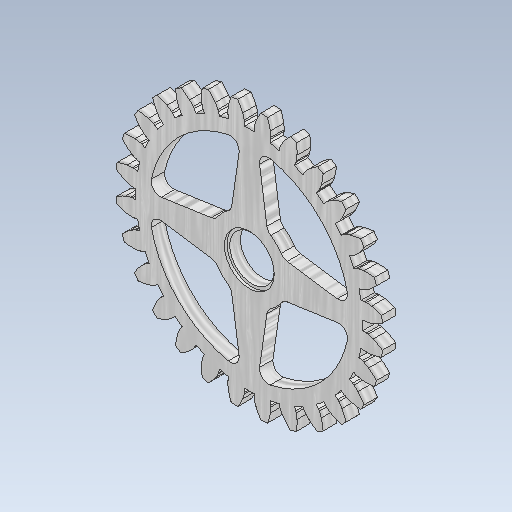
# Autodesk Inventor part: ｍ2歯数28ギア改二d10
Saved by Autodesk Inventor 2020.2 (Build 242310000, 310)
## iProperties
Created: 2020-02-11
Part Number: ｍ2歯数28ギア改二d10
Material: アルミニウム 7075
Document SubType Name: Modeling
Designer: aoyam
Density: 2.81 g/cm^3
Appearance: サテン - ブラシ仕上げ 重厚
Author: aoyam
Autodesk Inventor part; units mm, degrees
ref_plane "YZ Plane" through (0, 0, 0) normal (1, 0, 0) x (0, 1, 0)
ref_plane "XZ Plane" through (0, 0, 0) normal (0, 1, 0) x (-1, 0, 0)
ref_plane "XY Plane" through (0, 0, 0) normal (0, 0, 1) x (1, 0, 0)
sketch "スケッチ1" plane through (0, 0, 0) normal (0, 0, 1) x (1, 0, 0)
  arc A0 (149.6408, 131.6584) -> (149.5836, 131.2891) centre (152.0659, 131.0938) ccw
  arc A1 (150.0089, 132.8103) -> (149.6408, 131.6584) centre (156.3128, 130.1608) ccw
  arc A2 (151.1316, 134.8844) -> (150.0089, 132.8103) centre (160.8866, 128.2633) ccw
  arc A3 (147.4164, 131.2891) -> (147.3592, 131.6584) centre (144.9341, 131.0938) ccw
  arc A4 (147.3592, 131.6584) -> (146.9911, 132.8103) centre (140.6872, 130.1608) ccw
  arc A5 (146.9911, 132.8103) -> (145.8684, 134.8844) centre (136.1134, 128.2633) ccw
  arc A6 (149.5502, 130.4784) -> (147.4498, 130.4784) centre (148.5, 105) ccw
  arc A7 (145.8684, 134.8844) -> (144.4157, 134.7207) centre (148.5, 105) ccw
  line L0 (149.5502, 130.4784) -> (149.5836, 131.2891)
  line L1 (147.4498, 130.4784) -> (147.4164, 131.2891)
  line L2 (116.5, 105) -> (180.5, 105)
  line L3 (148.5, 73) -> (148.5, 137)
  line L4 (198.5, 135) -> (268.5, 135)
  line L5 (198.5, 127) -> (268.5, 127)
  line L6 (198.5, 119) -> (268.5, 119)
  line L7 (198.5, 111) -> (268.5, 111)
  line L8 (198.5, 103) -> (268.5, 103)
  line L9 (198.5, 95) -> (268.5, 95)
  line L10 (198.5, 87) -> (268.5, 87)
  line L11 (198.5, 79) -> (268.5, 79)
  line L12 (198.5, 71) -> (268.5, 71)
  line L13 (198.5, 63) -> (268.5, 63)
  line L14 (198.5, 55) -> (268.5, 55)
  line L15 (198.5, 47) -> (268.5, 47)
  line L16 (198.5, 39) -> (268.5, 39)
  line L17 (198.5, 135) -> (198.5, 39)
  line L18 (268.5, 135) -> (268.5, 39)
  line L19 (233.5, 127) -> (233.5, 39)
  arc A8 (144.4157, 134.7207) -> (143.7827, 132.4488) centre (155.3995, 130.4363) ccw
  arc A9 (143.7827, 132.4488) -> (143.6801, 131.2439) centre (150.5181, 131.2684) ccw
  arc A10 (143.6801, 131.2439) -> (143.7066, 130.8711) centre (146.1701, 131.2331) ccw
  line L20 (143.8544, 130.0733) -> (143.7066, 130.8711)
  arc A11 (143.8544, 130.0733) -> (141.8067, 129.6059) centre (148.5, 105) ccw
  line L21 (141.8067, 129.6059) -> (141.5937, 130.3888)
  arc A12 (141.5937, 130.3888) -> (141.4558, 130.7362) centre (139.217, 129.6461) ccw
  arc A13 (141.4558, 130.7362) -> (140.8405, 131.7773) centre (135.2843, 127.7914) ccw
  arc A14 (140.8405, 131.7773) -> (139.2845, 133.5495) centre (131.2474, 124.9238) ccw
  arc A15 (139.2845, 133.5495) -> (137.9046, 133.0667) centre (148.5, 105) ccw
  arc A16 (137.9046, 133.0667) -> (137.7931, 130.7109) centre (149.5664, 131.3339) ccw
  arc A17 (137.7931, 130.7109) -> (137.9612, 129.5133) centre (144.6222, 131.0589) ccw
  arc A18 (137.9612, 129.5133) -> (138.0699, 129.1558) centre (140.3911, 130.0569) ccw
  line L22 (138.3915, 128.4109) -> (138.0699, 129.1558)
  arc A19 (138.3915, 128.4109) -> (136.4992, 127.4996) centre (148.5, 105) ccw
  line L23 (136.4992, 127.4996) -> (136.1173, 128.2155)
  arc A20 (136.1173, 128.2155) -> (135.9056, 128.5234) centre (133.9655, 126.9625) ccw
  arc A21 (135.9056, 128.5234) -> (135.0741, 129.4015) centre (130.5441, 124.2792) ccw
  arc A22 (135.0741, 129.4015) -> (133.1627, 130.7831) centre (127.2465, 120.5852) ccw
  arc A23 (133.1627, 130.7831) -> (131.9249, 130.0053) centre (148.5, 105) ccw
  arc A24 (131.9249, 130.0053) -> (132.3403, 127.6838) centre (143.6798, 130.9109) ccw
  arc A25 (132.3403, 127.6838) -> (132.7707, 126.5536) centre (138.9208, 129.5427) ccw
  arc A26 (132.7707, 126.5536) -> (132.9562, 126.2292) centre (135.0187, 127.6243) ccw
  line L24 (133.4356, 125.5746) -> (132.9562, 126.2292)
  arc A27 (133.4356, 125.5746) -> (131.7934, 124.265) centre (148.5, 105) ccw
  line L25 (131.7934, 124.265) -> (131.2618, 124.878)
  arc A28 (131.2618, 124.878) -> (130.9869, 125.1311) centre (129.4428, 123.1776) ccw
  arc A29 (130.9869, 125.1311) -> (129.9808, 125.8022) centre (126.7042, 119.8003) ccw
  arc A30 (129.9808, 125.8022) -> (127.81, 126.7238) centre (124.3113, 115.4651) ccw
  arc A31 (127.81, 126.7238) -> (126.7762, 125.69) centre (148.5, 105) ccw
  arc A32 (126.7762, 125.69) -> (127.6978, 123.5192) centre (138.0349, 129.1887) ccw
  arc A33 (127.6978, 123.5192) -> (128.3689, 122.5131) centre (133.6997, 126.7958) ccw
  arc A34 (128.3689, 122.5131) -> (128.622, 122.2382) centre (130.3224, 124.0572) ccw
  line L26 (129.235, 121.7066) -> (128.622, 122.2382)
  arc A35 (129.235, 121.7066) -> (127.9254, 120.0644) centre (148.5, 105) ccw
  line L27 (127.9254, 120.0644) -> (127.2708, 120.5438)
  arc A36 (127.2708, 120.5438) -> (126.9464, 120.7293) centre (125.8757, 118.4813) ccw
  arc A37 (126.9464, 120.7293) -> (125.8162, 121.1597) centre (123.9573, 114.5792) ccw
  arc A38 (125.8162, 121.1597) -> (123.4947, 121.5751) centre (122.5891, 109.8202) ccw
  arc A39 (123.4947, 121.5751) -> (122.7169, 120.3373) centre (148.5, 105) ccw
  arc A40 (122.7169, 120.3373) -> (124.0985, 118.4259) centre (132.9148, 126.2535) ccw
  arc A41 (124.0985, 118.4259) -> (124.9766, 117.5944) centre (129.2208, 122.9559) ccw
  arc A42 (124.9766, 117.5944) -> (125.2845, 117.3827) centre (126.5375, 119.5345) ccw
  line L28 (126.0004, 117.0008) -> (125.2845, 117.3827)
  arc A43 (126.0004, 117.0008) -> (125.0891, 115.1085) centre (148.5, 105) ccw
  line L29 (125.0891, 115.1085) -> (124.3442, 115.4301)
  arc A44 (124.3442, 115.4301) -> (123.9867, 115.5388) centre (123.4431, 113.1089) ccw
  arc A45 (123.9867, 115.5388) -> (122.7891, 115.7069) centre (122.4411, 108.8778) ccw
  arc A46 (122.7891, 115.7069) -> (120.4333, 115.5954) centre (122.1661, 103.9336) ccw
  arc A47 (120.4333, 115.5954) -> (119.9505, 114.2155) centre (148.5, 105) ccw
  arc A48 (119.9505, 114.2155) -> (121.7227, 112.6595) centre (128.5762, 122.2526) ccw
  arc A49 (121.7227, 112.6595) -> (122.7638, 112.0442) centre (125.7086, 118.2157) ccw
  arc A50 (122.7638, 112.0442) -> (123.1112, 111.9063) centre (123.8539, 114.283) ccw
  line L30 (123.8941, 111.6933) -> (123.1112, 111.9063)
  arc A51 (123.8941, 111.6933) -> (123.4267, 109.6456) centre (148.5, 105) ccw
  line L31 (123.4267, 109.6456) -> (122.6289, 109.7934)
  arc A52 (122.6289, 109.7934) -> (122.2561, 109.8199) centre (122.2669, 107.3299) ccw
  arc A53 (122.2561, 109.8199) -> (121.0512, 109.7173) centre (122.2316, 102.9819) ccw
  arc A54 (121.0512, 109.7173) -> (118.7793, 109.0843) centre (123.0637, 98.1005) ccw
  arc A55 (118.7793, 109.0843) -> (118.6156, 107.6316) centre (148.5, 105) ccw
  arc A56 (118.6156, 107.6316) -> (120.6897, 106.5089) centre (125.2367, 117.3866) ccw
  arc A57 (120.6897, 106.5089) -> (121.8416, 106.1408) centre (123.3392, 112.8128) ccw
  arc A58 (121.8416, 106.1408) -> (122.2109, 106.0836) centre (122.4062, 108.5659) ccw
  line L32 (123.0216, 106.0502) -> (122.2109, 106.0836)
  arc A59 (123.0216, 106.0502) -> (123.0216, 103.9498) centre (148.5, 105) ccw
  line L33 (123.0216, 103.9498) -> (122.2109, 103.9164)
  arc A60 (122.2109, 103.9164) -> (121.8416, 103.8592) centre (122.4062, 101.4341) ccw
  arc A61 (121.8416, 103.8592) -> (120.6897, 103.4911) centre (123.3392, 97.1872) ccw
  arc A62 (120.6897, 103.4911) -> (118.6156, 102.3684) centre (125.2367, 92.6134) ccw
  arc A63 (118.6156, 102.3684) -> (118.7793, 100.9157) centre (148.5, 105) ccw
  arc A64 (118.7793, 100.9157) -> (121.0512, 100.2827) centre (123.0637, 111.8995) ccw
  arc A65 (121.0512, 100.2827) -> (122.2561, 100.1801) centre (122.2316, 107.0181) ccw
  arc A66 (122.2561, 100.1801) -> (122.6289, 100.2066) centre (122.2669, 102.6701) ccw
  line L34 (123.4267, 100.3544) -> (122.6289, 100.2066)
  arc A67 (123.4267, 100.3544) -> (123.8941, 98.3067) centre (148.5, 105) ccw
  line L35 (123.8941, 98.3067) -> (123.1112, 98.0937)
  arc A68 (123.1112, 98.0937) -> (122.7638, 97.9558) centre (123.8539, 95.717) ccw
  arc A69 (122.7638, 97.9558) -> (121.7227, 97.3405) centre (125.7086, 91.7843) ccw
  arc A70 (121.7227, 97.3405) -> (119.9505, 95.7845) centre (128.5762, 87.7474) ccw
  arc A71 (119.9505, 95.7845) -> (120.4333, 94.4046) centre (148.5, 105) ccw
  arc A72 (120.4333, 94.4046) -> (122.7891, 94.2931) centre (122.1661, 106.0664) ccw
  arc A73 (122.7891, 94.2931) -> (123.9867, 94.4612) centre (122.4411, 101.1222) ccw
  arc A74 (123.9867, 94.4612) -> (124.3442, 94.5699) centre (123.4431, 96.8911) ccw
  line L36 (125.0891, 94.8915) -> (124.3442, 94.5699)
  arc A75 (125.0891, 94.8915) -> (126.0004, 92.9992) centre (148.5, 105) ccw
  line L37 (126.0004, 92.9992) -> (125.2845, 92.6173)
  arc A76 (125.2845, 92.6173) -> (124.9766, 92.4056) centre (126.5375, 90.4655) ccw
  arc A77 (124.9766, 92.4056) -> (124.0985, 91.5741) centre (129.2208, 87.0441) ccw
  arc A78 (124.0985, 91.5741) -> (122.7169, 89.6627) centre (132.9148, 83.7465) ccw
  arc A79 (122.7169, 89.6627) -> (123.4947, 88.4249) centre (148.5, 105) ccw
  arc A80 (123.4947, 88.4249) -> (125.8162, 88.8403) centre (122.5891, 100.1798) ccw
  arc A81 (125.8162, 88.8403) -> (126.9464, 89.2707) centre (123.9573, 95.4208) ccw
  arc A82 (126.9464, 89.2707) -> (127.2708, 89.4562) centre (125.8757, 91.5187) ccw
  line L38 (127.9254, 89.9356) -> (127.2708, 89.4562)
  arc A83 (127.9254, 89.9356) -> (129.235, 88.2934) centre (148.5, 105) ccw
  line L39 (129.235, 88.2934) -> (128.622, 87.7618)
  arc A84 (128.622, 87.7618) -> (128.3689, 87.4869) centre (130.3224, 85.9428) ccw
  arc A85 (128.3689, 87.4869) -> (127.6978, 86.4808) centre (133.6997, 83.2042) ccw
  arc A86 (127.6978, 86.4808) -> (126.7762, 84.31) centre (138.0349, 80.8113) ccw
  arc A87 (126.7762, 84.31) -> (127.81, 83.2762) centre (148.5, 105) ccw
  arc A88 (127.81, 83.2762) -> (129.9808, 84.1978) centre (124.3113, 94.5349) ccw
  arc A89 (129.9808, 84.1978) -> (130.9869, 84.8689) centre (126.7042, 90.1997) ccw
  arc A90 (130.9869, 84.8689) -> (131.2618, 85.122) centre (129.4428, 86.8224) ccw
  line L40 (131.7934, 85.735) -> (131.2618, 85.122)
  arc A91 (131.7934, 85.735) -> (133.4356, 84.4254) centre (148.5, 105) ccw
  line L41 (133.4356, 84.4254) -> (132.9562, 83.7708)
  arc A92 (132.9562, 83.7708) -> (132.7707, 83.4464) centre (135.0187, 82.3757) ccw
  arc A93 (132.7707, 83.4464) -> (132.3403, 82.3162) centre (138.9208, 80.4573) ccw
  arc A94 (132.3403, 82.3162) -> (131.9249, 79.9947) centre (143.6798, 79.0891) ccw
  arc A95 (131.9249, 79.9947) -> (133.1627, 79.2169) centre (148.5, 105) ccw
  arc A96 (133.1627, 79.2169) -> (135.0741, 80.5985) centre (127.2465, 89.4148) ccw
  arc A97 (135.0741, 80.5985) -> (135.9056, 81.4766) centre (130.5441, 85.7208) ccw
  arc A98 (135.9056, 81.4766) -> (136.1173, 81.7845) centre (133.9655, 83.0375) ccw
  line L42 (136.4992, 82.5004) -> (136.1173, 81.7845)
  arc A99 (136.4992, 82.5004) -> (138.3915, 81.5891) centre (148.5, 105) ccw
  line L43 (138.3915, 81.5891) -> (138.0699, 80.8442)
  arc A100 (138.0699, 80.8442) -> (137.9612, 80.4867) centre (140.3911, 79.9431) ccw
  arc A101 (137.9612, 80.4867) -> (137.7931, 79.2891) centre (144.6222, 78.9411) ccw
  arc A102 (137.7931, 79.2891) -> (137.9046, 76.9333) centre (149.5664, 78.6661) ccw
  arc A103 (137.9046, 76.9333) -> (139.2845, 76.4505) centre (148.5, 105) ccw
  arc A104 (139.2845, 76.4505) -> (140.8405, 78.2227) centre (131.2474, 85.0762) ccw
  arc A105 (140.8405, 78.2227) -> (141.4558, 79.2638) centre (135.2843, 82.2086) ccw
  arc A106 (141.4558, 79.2638) -> (141.5937, 79.6112) centre (139.217, 80.3539) ccw
  line L44 (141.8067, 80.3941) -> (141.5937, 79.6112)
  arc A107 (141.8067, 80.3941) -> (143.8544, 79.9267) centre (148.5, 105) ccw
  line L45 (143.8544, 79.9267) -> (143.7066, 79.1289)
  arc A108 (143.7066, 79.1289) -> (143.6801, 78.7561) centre (146.1701, 78.7669) ccw
  arc A109 (143.6801, 78.7561) -> (143.7827, 77.5512) centre (150.5181, 78.7316) ccw
  arc A110 (143.7827, 77.5512) -> (144.4157, 75.2793) centre (155.3995, 79.5637) ccw
  arc A111 (144.4157, 75.2793) -> (145.8684, 75.1156) centre (148.5, 105) ccw
  arc A112 (145.8684, 75.1156) -> (146.9911, 77.1897) centre (136.1134, 81.7367) ccw
  arc A113 (146.9911, 77.1897) -> (147.3592, 78.3416) centre (140.6872, 79.8392) ccw
  arc A114 (147.3592, 78.3416) -> (147.4164, 78.7109) centre (144.9341, 78.9062) ccw
  line L46 (147.4498, 79.5216) -> (147.4164, 78.7109)
  arc A115 (147.4498, 79.5216) -> (149.5502, 79.5216) centre (148.5, 105) ccw
  line L47 (149.5502, 79.5216) -> (149.5836, 78.7109)
  arc A116 (149.5836, 78.7109) -> (149.6408, 78.3416) centre (152.0659, 78.9062) ccw
  arc A117 (149.6408, 78.3416) -> (150.0089, 77.1897) centre (156.3128, 79.8392) ccw
  arc A118 (150.0089, 77.1897) -> (151.1316, 75.1156) centre (160.8866, 81.7367) ccw
  arc A119 (151.1316, 75.1156) -> (152.5843, 75.2793) centre (148.5, 105) ccw
  arc A120 (152.5843, 75.2793) -> (153.2173, 77.5512) centre (141.6005, 79.5637) ccw
  arc A121 (153.2173, 77.5512) -> (153.3199, 78.7561) centre (146.4819, 78.7316) ccw
  arc A122 (153.3199, 78.7561) -> (153.2934, 79.1289) centre (150.8299, 78.7669) ccw
  line L48 (153.1456, 79.9267) -> (153.2934, 79.1289)
  arc A123 (153.1456, 79.9267) -> (155.1933, 80.3941) centre (148.5, 105) ccw
  line L49 (155.1933, 80.3941) -> (155.4063, 79.6112)
  arc A124 (155.4063, 79.6112) -> (155.5442, 79.2638) centre (157.783, 80.3539) ccw
  arc A125 (155.5442, 79.2638) -> (156.1595, 78.2227) centre (161.7157, 82.2086) ccw
  arc A126 (156.1595, 78.2227) -> (157.7155, 76.4505) centre (165.7526, 85.0762) ccw
  arc A127 (157.7155, 76.4505) -> (159.0954, 76.9333) centre (148.5, 105) ccw
  arc A128 (159.0954, 76.9333) -> (159.2069, 79.2891) centre (147.4336, 78.6661) ccw
  arc A129 (159.2069, 79.2891) -> (159.0388, 80.4867) centre (152.3778, 78.9411) ccw
  arc A130 (159.0388, 80.4867) -> (158.9301, 80.8442) centre (156.6089, 79.9431) ccw
  line L50 (158.6085, 81.5891) -> (158.9301, 80.8442)
  arc A131 (158.6085, 81.5891) -> (160.5008, 82.5004) centre (148.5, 105) ccw
  line L51 (160.5008, 82.5004) -> (160.8827, 81.7845)
  arc A132 (160.8827, 81.7845) -> (161.0944, 81.4766) centre (163.0345, 83.0375) ccw
  arc A133 (161.0944, 81.4766) -> (161.9259, 80.5985) centre (166.4559, 85.7208) ccw
  arc A134 (161.9259, 80.5985) -> (163.8373, 79.2169) centre (169.7535, 89.4148) ccw
  arc A135 (163.8373, 79.2169) -> (165.0751, 79.9947) centre (148.5, 105) ccw
  arc A136 (165.0751, 79.9947) -> (164.6597, 82.3162) centre (153.3202, 79.0891) ccw
  arc A137 (164.6597, 82.3162) -> (164.2293, 83.4464) centre (158.0792, 80.4573) ccw
  arc A138 (164.2293, 83.4464) -> (164.0438, 83.7708) centre (161.9813, 82.3757) ccw
  line L52 (163.5644, 84.4254) -> (164.0438, 83.7708)
  arc A139 (163.5644, 84.4254) -> (165.2066, 85.735) centre (148.5, 105) ccw
  line L53 (165.2066, 85.735) -> (165.7382, 85.122)
  arc A140 (165.7382, 85.122) -> (166.0131, 84.8689) centre (167.5572, 86.8224) ccw
  arc A141 (166.0131, 84.8689) -> (167.0192, 84.1978) centre (170.2958, 90.1997) ccw
  arc A142 (167.0192, 84.1978) -> (169.19, 83.2762) centre (172.6887, 94.5349) ccw
  arc A143 (169.19, 83.2762) -> (170.2238, 84.31) centre (148.5, 105) ccw
  arc A144 (170.2238, 84.31) -> (169.3022, 86.4808) centre (158.9651, 80.8113) ccw
  arc A145 (169.3022, 86.4808) -> (168.6311, 87.4869) centre (163.3003, 83.2042) ccw
  arc A146 (168.6311, 87.4869) -> (168.378, 87.7618) centre (166.6776, 85.9428) ccw
  line L54 (167.765, 88.2934) -> (168.378, 87.7618)
  arc A147 (167.765, 88.2934) -> (169.0746, 89.9356) centre (148.5, 105) ccw
  line L55 (169.0746, 89.9356) -> (169.7292, 89.4562)
  arc A148 (169.7292, 89.4562) -> (170.0536, 89.2707) centre (171.1243, 91.5187) ccw
  arc A149 (170.0536, 89.2707) -> (171.1838, 88.8403) centre (173.0427, 95.4208) ccw
  arc A150 (171.1838, 88.8403) -> (173.5053, 88.4249) centre (174.4109, 100.1798) ccw
  arc A151 (173.5053, 88.4249) -> (174.2831, 89.6627) centre (148.5, 105) ccw
  arc A152 (174.2831, 89.6627) -> (172.9015, 91.5741) centre (164.0852, 83.7465) ccw
  arc A153 (172.9015, 91.5741) -> (172.0234, 92.4056) centre (167.7792, 87.0441) ccw
  arc A154 (172.0234, 92.4056) -> (171.7155, 92.6173) centre (170.4625, 90.4655) ccw
  line L56 (170.9996, 92.9992) -> (171.7155, 92.6173)
  arc A155 (170.9996, 92.9992) -> (171.9109, 94.8915) centre (148.5, 105) ccw
  line L57 (171.9109, 94.8915) -> (172.6558, 94.5699)
  arc A156 (172.6558, 94.5699) -> (173.0133, 94.4612) centre (173.5569, 96.8911) ccw
  arc A157 (173.0133, 94.4612) -> (174.2109, 94.2931) centre (174.5589, 101.1222) ccw
  arc A158 (174.2109, 94.2931) -> (176.5667, 94.4046) centre (174.8339, 106.0664) ccw
  arc A159 (176.5667, 94.4046) -> (177.0495, 95.7845) centre (148.5, 105) ccw
  arc A160 (177.0495, 95.7845) -> (175.2773, 97.3405) centre (168.4238, 87.7474) ccw
  arc A161 (175.2773, 97.3405) -> (174.2362, 97.9558) centre (171.2914, 91.7843) ccw
  arc A162 (174.2362, 97.9558) -> (173.8888, 98.0937) centre (173.1461, 95.717) ccw
  line L58 (173.1059, 98.3067) -> (173.8888, 98.0937)
  arc A163 (173.1059, 98.3067) -> (173.5733, 100.3544) centre (148.5, 105) ccw
  line L59 (173.5733, 100.3544) -> (174.3711, 100.2066)
  arc A164 (174.3711, 100.2066) -> (174.7439, 100.1801) centre (174.7331, 102.6701) ccw
  arc A165 (174.7439, 100.1801) -> (175.9488, 100.2827) centre (174.7684, 107.0181) ccw
  arc A166 (175.9488, 100.2827) -> (178.2207, 100.9157) centre (173.9363, 111.8995) ccw
  arc A167 (178.2207, 100.9157) -> (178.3844, 102.3684) centre (148.5, 105) ccw
  arc A168 (178.3844, 102.3684) -> (176.3103, 103.4911) centre (171.7633, 92.6134) ccw
  arc A169 (176.3103, 103.4911) -> (175.1584, 103.8592) centre (173.6608, 97.1872) ccw
  arc A170 (175.1584, 103.8592) -> (174.7891, 103.9164) centre (174.5938, 101.4341) ccw
  line L60 (173.9784, 103.9498) -> (174.7891, 103.9164)
  arc A171 (173.9784, 103.9498) -> (173.9784, 106.0502) centre (148.5, 105) ccw
  line L61 (173.9784, 106.0502) -> (174.7891, 106.0836)
  arc A172 (174.7891, 106.0836) -> (175.1584, 106.1408) centre (174.5938, 108.5659) ccw
  arc A173 (175.1584, 106.1408) -> (176.3103, 106.5089) centre (173.6608, 112.8128) ccw
  arc A174 (176.3103, 106.5089) -> (178.3844, 107.6316) centre (171.7633, 117.3866) ccw
  arc A175 (178.3844, 107.6316) -> (178.2207, 109.0843) centre (148.5, 105) ccw
  arc A176 (178.2207, 109.0843) -> (175.9488, 109.7173) centre (173.9363, 98.1005) ccw
  arc A177 (175.9488, 109.7173) -> (174.7439, 109.8199) centre (174.7684, 102.9819) ccw
  arc A178 (174.7439, 109.8199) -> (174.3711, 109.7934) centre (174.7331, 107.3299) ccw
  line L62 (173.5733, 109.6456) -> (174.3711, 109.7934)
  arc A179 (173.5733, 109.6456) -> (173.1059, 111.6933) centre (148.5, 105) ccw
  line L63 (173.1059, 111.6933) -> (173.8888, 111.9063)
  arc A180 (173.8888, 111.9063) -> (174.2362, 112.0442) centre (173.1461, 114.283) ccw
  arc A181 (174.2362, 112.0442) -> (175.2773, 112.6595) centre (171.2914, 118.2157) ccw
  arc A182 (175.2773, 112.6595) -> (177.0495, 114.2155) centre (168.4238, 122.2526) ccw
  arc A183 (177.0495, 114.2155) -> (176.5667, 115.5954) centre (148.5, 105) ccw
  arc A184 (176.5667, 115.5954) -> (174.2109, 115.7069) centre (174.8339, 103.9336) ccw
  arc A185 (174.2109, 115.7069) -> (173.0133, 115.5388) centre (174.5589, 108.8778) ccw
  arc A186 (173.0133, 115.5388) -> (172.6558, 115.4301) centre (173.5569, 113.1089) ccw
  line L64 (171.9109, 115.1085) -> (172.6558, 115.4301)
  arc A187 (171.9109, 115.1085) -> (170.9996, 117.0008) centre (148.5, 105) ccw
  line L65 (170.9996, 117.0008) -> (171.7155, 117.3827)
  arc A188 (171.7155, 117.3827) -> (172.0234, 117.5944) centre (170.4625, 119.5345) ccw
  arc A189 (172.0234, 117.5944) -> (172.9015, 118.4259) centre (167.7792, 122.9559) ccw
  arc A190 (172.9015, 118.4259) -> (174.2831, 120.3373) centre (164.0852, 126.2535) ccw
  arc A191 (174.2831, 120.3373) -> (173.5053, 121.5751) centre (148.5, 105) ccw
  arc A192 (173.5053, 121.5751) -> (171.1838, 121.1597) centre (174.4109, 109.8202) ccw
  arc A193 (171.1838, 121.1597) -> (170.0536, 120.7293) centre (173.0427, 114.5792) ccw
  arc A194 (170.0536, 120.7293) -> (169.7292, 120.5438) centre (171.1243, 118.4813) ccw
  line L66 (169.0746, 120.0644) -> (169.7292, 120.5438)
  arc A195 (169.0746, 120.0644) -> (167.765, 121.7066) centre (148.5, 105) ccw
  line L67 (167.765, 121.7066) -> (168.378, 122.2382)
  arc A196 (168.378, 122.2382) -> (168.6311, 122.5131) centre (166.6776, 124.0572) ccw
  arc A197 (168.6311, 122.5131) -> (169.3022, 123.5192) centre (163.3003, 126.7958) ccw
  arc A198 (169.3022, 123.5192) -> (170.2238, 125.69) centre (158.9651, 129.1887) ccw
  arc A199 (170.2238, 125.69) -> (169.19, 126.7238) centre (148.5, 105) ccw
  arc A200 (169.19, 126.7238) -> (167.0192, 125.8022) centre (172.6887, 115.4651) ccw
  arc A201 (167.0192, 125.8022) -> (166.0131, 125.1311) centre (170.2958, 119.8003) ccw
  arc A202 (166.0131, 125.1311) -> (165.7382, 124.878) centre (167.5572, 123.1776) ccw
  line L68 (165.2066, 124.265) -> (165.7382, 124.878)
  arc A203 (165.2066, 124.265) -> (163.5644, 125.5746) centre (148.5, 105) ccw
  line L69 (163.5644, 125.5746) -> (164.0438, 126.2292)
  arc A204 (164.0438, 126.2292) -> (164.2293, 126.5536) centre (161.9813, 127.6243) ccw
  arc A205 (164.2293, 126.5536) -> (164.6597, 127.6838) centre (158.0792, 129.5427) ccw
  arc A206 (164.6597, 127.6838) -> (165.0751, 130.0053) centre (153.3202, 130.9109) ccw
  arc A207 (165.0751, 130.0053) -> (163.8373, 130.7831) centre (148.5, 105) ccw
  arc A208 (163.8373, 130.7831) -> (161.9259, 129.4015) centre (169.7535, 120.5852) ccw
  arc A209 (161.9259, 129.4015) -> (161.0944, 128.5234) centre (166.4559, 124.2792) ccw
  arc A210 (161.0944, 128.5234) -> (160.8827, 128.2155) centre (163.0345, 126.9625) ccw
  line L70 (160.5008, 127.4996) -> (160.8827, 128.2155)
  arc A211 (160.5008, 127.4996) -> (158.6085, 128.4109) centre (148.5, 105) ccw
  line L71 (158.6085, 128.4109) -> (158.9301, 129.1558)
  arc A212 (158.9301, 129.1558) -> (159.0388, 129.5133) centre (156.6089, 130.0569) ccw
  arc A213 (159.0388, 129.5133) -> (159.2069, 130.7109) centre (152.3778, 131.0589) ccw
  arc A214 (159.2069, 130.7109) -> (159.0954, 133.0667) centre (147.4336, 131.3339) ccw
  arc A215 (159.0954, 133.0667) -> (157.7155, 133.5495) centre (148.5, 105) ccw
  arc A216 (157.7155, 133.5495) -> (156.1595, 131.7773) centre (165.7526, 124.9238) ccw
  arc A217 (156.1595, 131.7773) -> (155.5442, 130.7362) centre (161.7157, 127.7914) ccw
  arc A218 (155.5442, 130.7362) -> (155.4063, 130.3888) centre (157.783, 129.6461) ccw
  line L72 (155.1933, 129.6059) -> (155.4063, 130.3888)
  arc A219 (155.1933, 129.6059) -> (153.1456, 130.0733) centre (148.5, 105) ccw
  line L73 (153.1456, 130.0733) -> (153.2934, 130.8711)
  arc A220 (153.2934, 130.8711) -> (153.3199, 131.2439) centre (150.8299, 131.2331) ccw
  arc A221 (153.3199, 131.2439) -> (153.2173, 132.4488) centre (146.4819, 131.2684) ccw
  arc A222 (153.2173, 132.4488) -> (152.5843, 134.7207) centre (141.6005, 130.4363) ccw
  arc A223 (152.5843, 134.7207) -> (151.1316, 134.8844) centre (148.5, 105) ccw
  circle A224 centre (148.5, 105) radius 5
  circle A225 centre (148.5, 105) radius 5.6
  arc A226 (143.6912, 112.1299) -> (153.3088, 112.1299) centre (148.5, 105) ccw
  circle A227 centre (148.5, 105) radius 25.5 construction
  arc A228 (143.8035, 127.0044) -> (153.1965, 127.0044) centre (148.5, 105) ccw
  line L74 (152.4482, 113.4984) -> (150.8001, 124.7588)
  circle A229 centre (148.5, 105) radius 25.5 construction
  line L75 (144.5518, 113.4984) -> (146.1999, 124.7588)
  arc A230 (146.1999, 124.7588) -> (143.8035, 127.0044) centre (144.221, 125.0484) ccw
  arc A231 (153.1965, 127.0044) -> (150.8001, 124.7588) centre (152.779, 125.0484) ccw
  arc A232 (152.4482, 113.4984) -> (153.3088, 112.1299) centre (154.4271, 113.788) ccw
  arc A233 (143.6912, 112.1299) -> (144.5518, 113.4984) centre (142.5729, 113.788) ccw
  line L76 (140.0016, 101.0518) -> (128.7412, 102.6999)
  arc A234 (141.3701, 100.1912) -> (140.0016, 101.0518) centre (139.712, 99.0729) ccw
  line L77 (140.0016, 108.9482) -> (128.7412, 107.3001)
  arc A235 (126.4956, 109.6965) -> (128.7412, 107.3001) centre (128.4516, 109.279) ccw
  arc A236 (140.0016, 108.9482) -> (141.3701, 109.8088) centre (139.712, 110.9271) ccw
  arc A237 (128.7412, 102.6999) -> (126.4956, 100.3035) centre (128.4516, 100.721) ccw
  line L78 (152.4482, 96.5016) -> (150.8001, 85.2412)
  arc A238 (153.3088, 97.8701) -> (152.4482, 96.5016) centre (154.4271, 96.212) ccw
  line L79 (144.5518, 96.5016) -> (146.1999, 85.2412)
  arc A239 (143.8035, 82.9956) -> (146.1999, 85.2412) centre (144.221, 84.9516) ccw
  arc A240 (144.5518, 96.5016) -> (143.6912, 97.8701) centre (142.5729, 96.212) ccw
  arc A241 (150.8001, 85.2412) -> (153.1965, 82.9956) centre (152.779, 84.9516) ccw
  line L80 (156.9984, 108.9482) -> (168.2588, 107.3001)
  arc A242 (155.6299, 109.8088) -> (156.9984, 108.9482) centre (157.288, 110.9271) ccw
  line L81 (156.9984, 101.0518) -> (168.2588, 102.6999)
  arc A243 (170.5044, 100.3035) -> (168.2588, 102.6999) centre (168.5484, 100.721) ccw
  arc A244 (156.9984, 101.0518) -> (155.6299, 100.1912) centre (157.288, 99.0729) ccw
  arc A245 (168.2588, 107.3001) -> (170.5044, 109.6965) centre (168.5484, 109.279) ccw
  point P0 (0, 0)
  point P1 (204.5, 129)
  point P2 (207, 121)
  point P3 (207, 113)
  point P4 (204.5, 105)
  point P5 (207, 97)
  point P6 (202, 89)
  point P7 (204.5, 81)
  point P8 (204.5, 73)
  point P9 (204.5, 65)
  point P10 (207, 57)
  point P11 (207, 49)
  point P12 (204.5, 41)
  point P13 (234.5, 121)
  point P14 (249.5, 113)
  point P15 (250.75, 105)
  point P16 (247, 97)
  point P17 (249.5, 89)
  point P18 (243.25, 81)
  point P19 (249.5, 73)
  point P20 (249.5, 65)
  point P21 (244.5, 57)
  point P22 (252, 49)
  point P23 (252, 41)
  point P24 (149.5, 150.5)
  point P25 (149.5, 144.5)
  point P26 (165.6875, 150.5)
  point P27 (168.875, 144.5)
  point P28 (141.3793, 136.1977)
  point P29 (134.6157, 133.831)
  point P30 (128.5483, 130.0186)
  point P31 (123.4814, 124.9517)
  point P32 (119.669, 118.8843)
  point P33 (117.3023, 112.1207)
  point P34 (116.5, 105)
  point P35 (117.3023, 97.8793)
  point P36 (119.669, 91.1157)
  point P37 (123.4814, 85.0483)
  point P38 (128.5483, 79.9814)
  point P39 (134.6157, 76.169)
  point P40 (141.3793, 73.8023)
  point P41 (155.6207, 73.8023)
  point P42 (162.3843, 76.169)
  point P43 (168.4517, 79.9814)
  point P44 (173.5186, 85.0483)
  point P45 (177.331, 91.1157)
  point P46 (179.6977, 97.8793)
  point P47 (180.5, 105)
  point P48 (179.6977, 112.1207)
  point P49 (177.331, 118.8843)
  point P50 (173.5186, 124.9517)
  point P51 (168.4517, 130.0186)
  point P52 (162.3843, 133.831)
  point P53 (155.6207, 136.1977)
  point P54 (173.9784, 106.0502)
  point P55 (176.3103, 106.5089)
  point P56 (175.9488, 109.7173)
  point P57 (174.7439, 109.8199)
  point P58 (174.2362, 112.0442)
  point P59 (177.0495, 114.2155)
  point P60 (171.7155, 117.3827)
  point P61 (172.9015, 118.4259)
  point P62 (174.2831, 120.3373)
  point P63 (173.5053, 121.5751)
  point P64 (169.7292, 120.5438)
  point P65 (168.6311, 122.5131)
  point P66 (170.2238, 125.69)
  point P67 (169.19, 126.7238)
  point P68 (167.0192, 125.8022)
  point P69 (166.0131, 125.1311)
  point P70 (163.5644, 125.5746)
  point P71 (163.8373, 130.7831)
  point P72 (158.9301, 129.1558)
  point P73 (159.0388, 129.5133)
  point P74 (159.2069, 130.7109)
  point P75 (159.0954, 133.0667)
  point P76 (157.7155, 133.5495)
  point P77 (155.5442, 130.7362)
  point P78 (155.1933, 129.6059)
  point P79 (153.1456, 130.0733)
  point P80 (153.2934, 130.8711)
  point P81 (153.2173, 132.4488)
  point P82 (152.5843, 134.7207)
  point P83 (149.5836, 131.2891)
  point P84 (147.4498, 130.4784)
  point P85 (147.3592, 131.6584)
  point P86 (145.8684, 134.8844)
  point P87 (144.4157, 134.7207)
  point P88 (143.7827, 132.4488)
  point P89 (141.4558, 130.7362)
  point P90 (140.8405, 131.7773)
  point P91 (137.9046, 133.0667)
  point P92 (137.9612, 129.5133)
  point P93 (133.1627, 130.7831)
  point P94 (131.9249, 130.0053)
  point P95 (132.3403, 127.6838)
  point P96 (132.7707, 126.5536)
  point P97 (131.2618, 124.878)
  point P98 (127.81, 126.7238)
  point P99 (126.7762, 125.69)
  point P100 (127.6978, 123.5192)
  point P101 (128.3689, 122.5131)
  point P102 (127.9254, 120.0644)
  point P103 (127.2708, 120.5438)
  point P104 (126.9464, 120.7293)
  point P105 (123.4947, 121.5751)
  point P106 (122.7169, 120.3373)
  point P107 (124.9766, 117.5944)
  point P108 (123.9867, 115.5388)
  point P109 (122.7891, 115.7069)
  point P110 (120.4333, 115.5954)
  point P111 (119.9505, 114.2155)
  point P112 (121.7227, 112.6595)
  point P113 (122.7638, 112.0442)
  point P114 (122.6289, 109.7934)
  point P115 (122.2561, 109.8199)
  point P116 (121.0512, 109.7173)
  point P117 (120.6897, 106.5089)
  point P118 (123.0216, 106.0502)
  point P119 (123.0216, 103.9498)
  point P120 (121.8416, 103.8592)
  point P121 (120.6897, 103.4911)
  point P122 (118.7793, 100.9157)
  point P123 (122.2561, 100.1801)
  point P124 (123.4267, 100.3544)
  point P125 (121.7227, 97.3405)
  point P126 (120.4333, 94.4046)
  point P127 (122.7891, 94.2931)
  point P128 (123.9867, 94.4612)
  point P129 (126.0004, 92.9992)
  point P130 (124.9766, 92.4056)
  point P131 (125.8162, 88.8403)
  point P132 (126.9464, 89.2707)
  point P133 (127.6978, 86.4808)
  point P134 (126.7762, 84.31)
  point P135 (127.81, 83.2762)
  point P136 (129.9808, 84.1978)
  point P137 (130.9869, 84.8689)
  point P138 (131.2618, 85.122)
  point P139 (133.4356, 84.4254)
  point P140 (132.7707, 83.4464)
  point P141 (133.1627, 79.2169)
  point P142 (135.0741, 80.5985)
  point P143 (135.9056, 81.4766)
  point P144 (136.1173, 81.7845)
  point P145 (137.9612, 80.4867)
  point P146 (137.9046, 76.9333)
  point P147 (140.8405, 78.2227)
  point P148 (141.5937, 79.6112)
  point P149 (141.8067, 80.3941)
  point P150 (143.6801, 78.7561)
  point P151 (143.7827, 77.5512)
  point P152 (144.4157, 75.2793)
  point P153 (145.8684, 75.1156)
  point P154 (146.9911, 77.1897)
  point P155 (147.3592, 78.3416)
  point P156 (147.4498, 79.5216)
  point P157 (149.5502, 79.5216)
  point P158 (149.5836, 78.7109)
  point P159 (150.0089, 77.1897)
  point P160 (151.1316, 75.1156)
  point P161 (153.2173, 77.5512)
  point P162 (153.3199, 78.7561)
  point P163 (153.1456, 79.9267)
  point P164 (157.7155, 76.4505)
  point P165 (159.2069, 79.2891)
  point P166 (160.5008, 82.5004)
  point P167 (161.0944, 81.4766)
  point P168 (161.9259, 80.5985)
  point P169 (164.2293, 83.4464)
  point P170 (165.2066, 85.735)
  point P171 (165.7382, 85.122)
  point P172 (166.0131, 84.8689)
  point P173 (169.19, 83.2762)
  point P174 (170.2238, 84.31)
  point P175 (169.3022, 86.4808)
  point P176 (168.6311, 87.4869)
  point P177 (170.0536, 89.2707)
  point P178 (174.2831, 89.6627)
  point P179 (172.9015, 91.5741)
  point P180 (172.0234, 92.4056)
  point P181 (173.0133, 94.4612)
  point P182 (174.2109, 94.2931)
  point P183 (176.5667, 94.4046)
  point P184 (177.0495, 95.7845)
  point P185 (174.2362, 97.9558)
  point P186 (173.5733, 100.3544)
  point P187 (174.3711, 100.2066)
  point P188 (174.7439, 100.1801)
  point P189 (178.2207, 100.9157)
  point P190 (176.3103, 103.4911)
  point P191 (150.4108, 127.4187)
  point P192 (144.4157, 112.5683)
  point P193 (146.5892, 127.4187)
  point P194 (152.5843, 112.5683)
  point P195 (126.0813, 106.9108)
  point P196 (126.0813, 103.0892)
  point P197 (140.9317, 100.9157)
  point P198 (140.9317, 109.0843)
  point P199 (146.5892, 82.5813)
  dimension "d2" = 360
  dimension "d4" = 10
  dimension "d7" = 0.6
  dimension "d10" = 3
  dimension "d11" = 3
  dimension "d12" = 2
  dimension "d15" = 360
  constraints: 488 point on circle, 246 centre point, 164 end point, 16 point on line, 8 tangent, 4 coincident, 3 equal radius, 2 symmetric about line, 1208 other
  measures "d4" diameter of A224
  measures "d7" radial gap between concentric circles of A224 A225
  measures "d10" radial gap between concentric circles of A225 A226
  measures "d11" radial gap between concentric circles of A227 A228
  measures "d12" radius of A230
extrude "押し出し1" add sketch "スケッチ1" along normal blind 3 contours A1 A2 A223 A222 A221 A220 L73 A219 L72 A218 A217 A216 A215 A214 A213 A212 L71 A211 L70 A210 A209 A208 A207 A206 A205 A204 L69 A203 L68 A202 A201 A200 A199 A198 A197 A196 L67 A195 L66 A194 A193 A192 A191 A190 A189 A188 L65 A187 L64 A186 A185 A184 A183 A182 A181 A180 L63 A179 L62 A178 A177 A176 A175 A174 A173 A172 L61 A171 L2 A228 A231 L74 A232 A226 A225 L3 A6 L0 A0 | L3 A225 L2 A226 A233 L75 A230 A228 A59 L32 A58 A57 A56 A55 A54 A53 A52 L31 A51 L30 A50 A49 A48 A47 A46 A45 A44 L29 A43 L28 A42 A41 A40 A39 A38 A37 A36 L27 A35 L26 A34 A33 A32 A31 A30 A29 A28 L25 A27 L24 A26 A25 A24 A23 A22 A21 A20 L23 A19 L22 A18 A17 A16 A15 A14 A13 A12 L21 A11 L20 A10 A9 A8 A7 A5 A4 A3 L1 A6 | L2 A226 L3 A225 | A225 L3 A226 L2 | A226 A242 L80 A245 A228 L2 | L2 A228 A243 L81 A244 A226 | A226 A234 L76 A237 A228 L2 | L2 A228 A235 L77 A236 A226 | L2 A171 L60 A170 A169 A168 A167 A166 A165 A164 L59 A163 L58 A162 A161 A160 A159 A158 A157 A156 L57 A155 L56 A154 A153 A152 A151 A150 A149 A148 L55 A147 L54 A146 A145 A144 A143 A142 A141 A140 L53 A139 L52 A138 A137 A136 A135 A134 A133 A132 L51 A131 L50 A130 A129 A128 A127 A126 A125 A124 L49 A123 L48 A122 A121 A120 A119 A118 A117 A116 L47 A115 L3 A228 | A226 A238 L78 A241 A228 L3 | L3 A228 A239 L79 A240 A226 | A228 L3 A115 L46 A114 A113 A112 A111 A110 A109 A108 L45 A107 L44 A106 A105 A104 A103 A102 A101 A100 L43 A99 L42 A98 A97 A96 A95 A94 A93 A92 L41 A91 L40 A90 A89 A88 A87 A86 A85 A84 L39 A83 L38 A82 A81 A80 A79 A78 A77 A76 L37 A75 L36 A74 A73 A72 A71 A70 A69 A68 L35 A67 L34 A66 A65 A64 A63 A62 A61 A60 L33 A59 L2
extrude "押し出し2" add sketch "スケッチ1" along normal blind 2.4 contours A225 L2 A224 L3 | L3 A224 L2 A225 | A225 L3 A224 L2 | L2 A224 L3 A225
